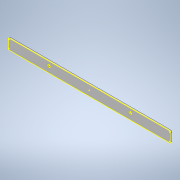
# Autodesk Inventor part: DisplayAcrylicHolder
Saved by Autodesk Inventor 2022 (Build 260153000, 153)
## iProperties
Created: 2021-04-23
Part Number: DisplayAcrylicHolder
Material: Generic
Document SubType Name: Modeling
Designer: Viktor
Density: 1 g/cm^3
Appearance: Default
Author: Viktor
Autodesk Inventor part; units mm, degrees
ref_plane "YZ Plane" through (0, 0, 0) normal (1, 0, 0) x (0, 1, 0)
ref_plane "XZ Plane" through (0, 0, 0) normal (0, 1, 0) x (-1, 0, 0)
ref_plane "XY Plane" through (0, 0, 0) normal (0, 0, 1) x (1, 0, 0)
sketch "Sketch1" plane through (0, 0, 0) normal (0, 0, 1) x (1, 0, 0)
  line L0 (-140, -9) -> (140, -9)
  line L1 (140, -9) -> (140, 9)
  line L2 (140, 9) -> (-140, 9)
  line L3 (-140, 9) -> (-140, -9)
  line L4 (-140, -9) -> (140, 9) construction
  line L5 (140, -9) -> (-140, 9) construction
  point P0 (0, 0)
  dimension "d0" = 280
  dimension "d1" = 18
  constraints: 12 end point, 2 midpoint, 2 parallel, 1 horizontal, 1 perpendicular
  measures "d0" distance of L1.end L2.end
  measures "d1" distance between parallel lines of L2 L0
extrude "Extrusion1" add sketch "Sketch1" along normal blind 2
sketch "Sketch3" plane through (0, 0, 2) normal (0, 0, 1) x (1, 0, 0)
  line L0 (-99.5384, 1.5) -> (103.3668, 1.5) construction
  circle A0 centre (-70, 1.5) radius 2.25
  circle A1 centre (70, 1.5) radius 2.25
  line L1 (140, 9) -> (-140, 9) projected
  line L2 (-108, -2.5) -> (123, -2.5) construction
  line L3 (-140, -9) -> (140, -9) projected
  point P0 (0, 0)
  dimension "d4" = 4.5
  dimension "d5" = 4.5
  dimension "d6" = 7.5
  dimension "d7" = 6.5
  dimension "d8" = 70
  dimension "d9" = 70
  constraints: 4 end point, 2 centre point, 2 horizontal, 2 point on line
  measures "d4" diameter of A0
  measures "d5" diameter of A1
  measures "d6" distance between parallel lines of L1 L0
  measures "d7" distance between parallel lines of L3 L2
  measures "d8" horizontal distance of point (0, 0) A0.centre
  measures "d9" horizontal distance of point (0, 0) A1.centre
extrude "Extrusion2" cut sketch "Sketch3" against normal blind 2
fillet "Fillet1" radius 2 4 edges at (-140, 9, 1) (-140, -9, 1) (140, 9, 1) (140, -9, 1)
sketch "Sketch4" plane through (0, 0, 2) normal (0, 0, 1) x (1, 0, 0)
  arc A0 (138, -9) -> (140, -7) centre (138, -7) ccw projected
  line L0 (140, -7) -> (140, 7) projected
  arc A1 (140, 7) -> (138, 9) centre (138, 7) ccw projected
  line L1 (138, 9) -> (-138, 9) projected
  arc A2 (-138, 9) -> (-140, 7) centre (-138, 7) ccw projected
  line L2 (-140, 7) -> (-140, -7) projected
  arc A3 (-140, -7) -> (-138, -9) centre (-138, -7) ccw projected
  line L3 (-138, -9) -> (138, -9) projected
  circle A4 centre (70, 1.5) radius 2.25 projected
  circle A5 centre (-70, 1.5) radius 2.25 projected
  point P0 (0, 0)
equation "\"d5\" = d4"
equation "\"d9\" = d8"
body "Solid1"
